Autodesk Fusion 360 part; units mm, degrees
note: some values were not read from the file. Set by a fixed rule: which sketch regions a step uses.
(part 2 of 6)
  line L1001 (386, 233.1906) -> (388, 234.3453)
  line L1002 (350.25, 210.9537) -> (352.25, 212.1084)
  line L1003 (360.5, 236.6547) -> (358.5, 237.8094)
  line L1004 (360.5, 236.6547) -> (358.5, 237.8094)
  line L1005 (378.5, 218.6547) -> (378.5, 216.3453)
  line L1006 (378.5, 245.6547) -> (378.5, 243.3453)
  line L1007 (378.5, 216.3453) -> (380.5, 215.1906)
  line L1008 (350.25, 206.5725) -> (348.25, 205.4178)
  line L1009 (355, 234.3453) -> (355, 236.6547)
  line L1010 (382.5, 243.3453) -> (382.5, 245.6547)
  line L1011 (391.5, 237.8094) -> (389.5, 236.6547)
  line L1012 (362, 236.6547) -> (362, 234.3453)
  line L1013 (388.75, 237.9537) -> (390.75, 239.1084)
  line L1014 (345.5, 207.3453) -> (347.5, 206.1906)
  line L1015 (379.75, 250.4178) -> (377.75, 251.5725)
  line L1016 (388.75, 233.5725) -> (386.75, 232.4178)
  line L1017 (347.5, 210.8094) -> (345.5, 209.6547)
  line L1018 (362, 236.6547) -> (362, 234.3453)
  line L1019 (377, 243.3453) -> (377, 245.6547)
  line L1020 (388, 236.6547) -> (386, 237.8094)
  line L1021 (381.25, 232.4178) -> (381.25, 230.1084)
  line L1022 (366, 227.6547) -> (364, 228.8094)
  line L1023 (382.5, 216.3453) -> (382.5, 218.6547)
  line L1024 (378.5, 245.6547) -> (378.5, 243.3453)
  line L1025 (388, 236.6547) -> (386, 237.8094)
  line L1026 (377, 243.3453) -> (377, 245.6547)
  line L1027 (358.5, 233.1906) -> (360.5, 234.3453)
  line L1028 (358.5, 237.8094) -> (356.5, 236.6547)
  line L1029 (389.5, 234.3453) -> (391.5, 233.1906)
  line L1030 (378.5, 243.3453) -> (380.5, 242.1906)
  line L1031 (382.5, 245.6547) -> (380.5, 246.8094)
  line L1032 (389.5, 234.3453) -> (391.5, 233.1906)
  line L1033 (350.25, 210.9537) -> (352.25, 212.1084)
  line L1034 (366.75, 224.5725) -> (364.75, 223.4178)
  line L1035 (358.5, 237.8094) -> (356.5, 236.6547)
  line L1036 (379.75, 241.4178) -> (377.75, 242.5725)
  line L1037 (388, 234.3453) -> (388, 236.6547)
  line L1038 (363.25, 230.1084) -> (363.25, 232.4178)
  line L1039 (351, 216.3453) -> (353, 215.1906)
  line L1040 (382.5, 245.6547) -> (380.5, 246.8094)
  line L1041 (359.25, 239.1084) -> (361.25, 237.9537)
  line L1042 (378.5436, 252.3202) -> (380.5, 251.1906)
  arc A23 (381.6602, 251.8605) -> (378.5436, 252.3202) centre (375, 217.5) ccw
  line L1043 (378.5436, 252.3202) -> (380.5, 251.1906)
  line L1044 (349.5, 216.3453) -> (349.5, 218.6547)
  line L1045 (377.75, 242.5725) -> (375.75, 241.4178)
  line L1046 (369.5, 237.8094) -> (367.5, 236.6547)
  line L1047 (380.5, 251.1906) -> (381.6602, 251.8605)
  line L1048 (375.75, 248.1084) -> (377.75, 246.9537)
  line L1049 (364.75, 239.1084) -> (366.75, 237.9537)
  line L1050 (367.5, 234.3453) -> (369.5, 233.1906)
  line L1051 (345.5, 209.6547) -> (345.5, 207.3453)
  line L1052 (347.5, 206.1906) -> (349.5, 207.3453)
  line L1053 (353.75, 239.1084) -> (355.75, 237.9537)
  line L1054 (375.75, 248.1084) -> (377.75, 246.9537)
  line L1055 (380.5, 246.8094) -> (378.5, 245.6547)
  line L1056 (353, 210.8094) -> (351, 209.6547)
  line L1057 (364, 233.1906) -> (366, 234.3453)
  line L1058 (356.5, 234.3453) -> (358.5, 233.1906)
  line L1059 (366.75, 242.5725) -> (364.75, 241.4178)
  line L1060 (368.75, 230.1084) -> (368.75, 232.4178)
  line L1061 (368.75, 230.1084) -> (368.75, 232.4178)
  line L1062 (366.75, 237.9537) -> (368.75, 239.1084)
  line L1063 (368.75, 232.4178) -> (366.75, 233.5725)
  line L1064 (353, 219.8094) -> (351, 218.6547)
  line L1065 (380.5, 242.1906) -> (382.5, 243.3453)
  line L1066 (360.5, 234.3453) -> (360.5, 236.6547)
  line L1067 (369.5, 228.8094) -> (367.5, 227.6547)
  line L1068 (348.25, 212.1084) -> (350.25, 210.9537)
  line L1069 (355.75, 237.9537) -> (357.75, 239.1084)
  line L1070 (390.75, 232.4178) -> (388.75, 233.5725)
  line L1071 (345.5, 218.6547) -> (345.5, 216.3453)
  line L1072 (367.5, 225.3453) -> (369.5, 224.1906)
  line L1073 (377.75, 251.5725) -> (375.75, 250.4178)
  line L1074 (368.75, 223.4178) -> (366.75, 224.5725)
  line L1075 (366, 236.6547) -> (364, 237.8094)
  line L1076 (390.75, 232.4178) -> (388.75, 233.5725)
  line L1077 (384, 234.3453) -> (386, 233.1906)
  line L1078 (346.75, 205.4178) -> (344.75, 206.5725)
  line L1079 (366.75, 237.9537) -> (368.75, 239.1084)
  line L1080 (350.25, 219.9537) -> (352.25, 221.1084)
  line L1081 (356.5, 236.6547) -> (356.5, 234.3453)
  line L1082 (366, 227.6547) -> (364, 228.8094)
  line L1083 (377.75, 242.5725) -> (375.75, 241.4178)
  line L1084 (352.25, 214.4178) -> (350.25, 215.5725)
  line L1085 (345.5, 216.3453) -> (347.5, 215.1906)
  line L1086 (361.25, 233.5725) -> (359.25, 232.4178)
  line L1087 (352.25, 214.4178) -> (350.25, 215.5725)
  line L1088 (352.25, 205.4178) -> (350.25, 206.5725)
  line L1089 (369.5, 237.8094) -> (367.5, 236.6547)
  line L1090 (360.5, 234.3453) -> (360.5, 236.6547)
  line L1091 (388.75, 237.9537) -> (390.75, 239.1084)
  line L1092 (364.75, 223.4178) -> (364.75, 221.1084)
  line L1093 (385.25, 241.4178) -> (383.25, 242.5725)
  line L1094 (349.5, 216.3453) -> (349.5, 218.6547)
  line L1095 (364, 242.1906) -> (366, 243.3453)
  line L1096 (366.75, 228.9537) -> (368.75, 230.1084)
  line L1097 (347.5, 219.8094) -> (345.5, 218.6547)
  line L1098 (364.75, 241.4178) -> (364.75, 239.1084)
  line L1099 (379.75, 250.4178) -> (377.75, 251.5725)
  line L1100 (368.75, 239.1084) -> (368.75, 241.4178)
  line L1101 (380.5, 237.8094) -> (378.5, 236.6547)
  line L1102 (345.5, 218.6547) -> (345.5, 216.3453)
  line L1103 (367.5, 234.3453) -> (369.5, 233.1906)
  line L1104 (347.5, 219.8094) -> (345.5, 218.6547)
  line L1105 (385.25, 241.4178) -> (383.25, 242.5725)
  line L1106 (366, 236.6547) -> (364, 237.8094)
  line L1107 (357.75, 239.1084) -> (357.75, 241.4178)
  line L1108 (357.75, 230.1084) -> (357.75, 232.4178)
  line L1109 (363.25, 239.1084) -> (363.25, 241.4178)
  line L1110 (346.75, 214.4178) -> (344.75, 215.5725)
  line L1111 (383.25, 242.5725) -> (381.25, 241.4178)
  line L1112 (367.5, 243.3453) -> (369.5, 242.1906)
  line L1113 (351, 216.3453) -> (353, 215.1906)
  line L1114 (369.5, 228.8094) -> (367.5, 227.6547)
  line L1115 (366.75, 228.9537) -> (368.75, 230.1084)
  line L1116 (368.75, 241.4178) -> (366.75, 242.5725)
  line L1117 (380.5, 233.1906) -> (382.5, 234.3453)
  line L1118 (377.75, 251.5725) -> (375.75, 250.4178)
  line L1119 (367.5, 225.3453) -> (369.5, 224.1906)
  line L1120 (347.5, 215.1906) -> (349.5, 216.3453)
  arc A24 (390.75, 248.756) -> (386.8045, 250.4493) centre (375, 217.5) ccw
  line L1121 (344.75, 219.9537) -> (346.75, 221.1084)
  line L1122 (347.5, 215.1906) -> (349.5, 216.3453)
  line L1123 (363.25, 239.1084) -> (363.25, 241.4178)
  line L1124 (364.75, 230.1084) -> (366.75, 228.9537)
  line L1125 (359.25, 232.4178) -> (359.25, 230.1084)
  line L1126 (359.25, 232.4178) -> (359.25, 230.1084)
  line L1127 (350.25, 215.5725) -> (348.25, 214.4178)
  line L1128 (353.75, 232.4178) -> (353.75, 230.1084)
  line L1129 (356.5, 236.6547) -> (356.5, 234.3453)
  line L1130 (377.75, 237.9537) -> (379.75, 239.1084)
  line L1131 (359.25, 241.4178) -> (359.25, 239.1084)
  line L1132 (383.25, 242.5725) -> (381.25, 241.4178)
  line L1133 (349.5, 218.6547) -> (347.5, 219.8094)
  line L1134 (363.25, 221.1084) -> (363.25, 223.4178)
  line L1135 (364.75, 232.4178) -> (364.75, 230.1084)
  line L1136 (350.25, 215.5725) -> (348.25, 214.4178)
  line L1137 (381.25, 232.4178) -> (381.25, 230.1084)
  line L1138 (364, 224.1906) -> (366, 225.3453)
  line L1139 (344.75, 219.9537) -> (346.75, 221.1084)
  line L1140 (366.75, 224.5725) -> (364.75, 223.4178)
  line L1141 (364.75, 241.4178) -> (364.75, 239.1084)
  line L1142 (377, 252.3453) -> (377, 252.4428)
  line L1143 (367.5, 245.6547) -> (367.5, 243.3453)
  line L1144 (353.75, 232.4178) -> (353.75, 230.1084)
  arc A25 (381.6602, 251.8605) -> (378.5436, 252.3202) centre (375, 217.5) ccw
  line L1145 (366.75, 242.5725) -> (364.75, 241.4178)
  line L1146 (357.75, 230.1084) -> (357.75, 232.4178)
  line L1147 (366.75, 233.5725) -> (364.75, 232.4178)
  line L1148 (348.25, 221.1084) -> (350.25, 219.9537)
  line L1149 (386.8045, 250.4493) -> (386.75, 250.4178)
  line L1150 (368.75, 241.4178) -> (366.75, 242.5725)
  line L1151 (377, 234.3453) -> (377, 236.6547)
  line L1152 (368.75, 239.1084) -> (368.75, 241.4178)
  line L1153 (375.75, 239.1084) -> (377.75, 237.9537)
  line L1154 (346.75, 223.4178) -> (344.75, 224.5725)
  line L1155 (367.5, 245.6547) -> (367.5, 243.3453)
  line L1156 (364.75, 250.4178) -> (364.75, 248.1084)
  line L1157 (363.25, 230.1084) -> (363.25, 232.4178)
  line L1158 (350.25, 219.9537) -> (352.25, 221.1084)
  line L1159 (355, 236.6547) -> (353, 237.8094)
  line L1160 (377.75, 233.5725) -> (375.75, 232.4178)
  line L1161 (364.75, 239.1084) -> (366.75, 237.9537)
  line L1162 (355, 236.6547) -> (353, 237.8094)
  line L1163 (368.75, 221.1084) -> (368.75, 223.4178)
  line L1164 (390.75, 230.1084) -> (390.75, 232.4178)
  line L1165 (366, 243.3453) -> (366, 245.6547)
  line L1166 (378.5, 236.6547) -> (378.5, 234.3453)
  line L1167 (364.75, 232.4178) -> (364.75, 230.1084)
  line L1168 (348.25, 221.1084) -> (350.25, 219.9537)
  line L1169 (353, 219.8094) -> (351, 218.6547)
  line L1170 (353, 233.1906) -> (355, 234.3453)
  line L1171 (351, 218.6547) -> (351, 216.3453)
  line L1172 (355, 227.6547) -> (353, 228.8094)
  line L1173 (368.75, 223.4178) -> (366.75, 224.5725)
  line L1174 (351, 218.6547) -> (351, 216.3453)
  line L1175 (377.75, 233.5725) -> (375.75, 232.4178)
  line L1176 (345.5, 216.3453) -> (347.5, 215.1906)
  line L1177 (359.25, 248.756) -> (359.25, 248.1084)
  line L1178 (366, 225.3453) -> (366, 227.6547)
  line L1179 (380.5, 233.1906) -> (382.5, 234.3453)
  line L1180 (348.25, 230.1084) -> (350.25, 228.9537)
  line L1181 (359.25, 248.756) -> (359.25, 248.1084)
  line L1182 (377, 234.3453) -> (377, 236.6547)
  line L1183 (380.5, 251.1906) -> (381.6602, 251.8605)
  line L1184 (368.75, 248.1084) -> (368.75, 250.4178)
  line L1185 (382.5, 236.6547) -> (380.5, 237.8094)
  line L1186 (346.75, 214.4178) -> (344.75, 215.5725)
  line L1187 (383.25, 237.9537) -> (385.25, 239.1084)
  line L1188 (353, 224.1906) -> (355, 225.3453)
  line L1189 (377.75, 237.9537) -> (379.75, 239.1084)
  line L1190 (364, 233.1906) -> (366, 234.3453)
  line L1191 (382.5, 234.3453) -> (382.5, 236.6547)
  line L1192 (366, 243.3453) -> (366, 245.6547)
  line L1193 (366.75, 233.5725) -> (364.75, 232.4178)
  line L1194 (375.75, 232.4178) -> (375.75, 230.1084)
  line L1195 (364.75, 230.1084) -> (366.75, 228.9537)
  line L1196 (368.3398, 251.8605) -> (369.5, 251.1906)
  line L1197 (364, 242.1906) -> (366, 243.3453)
  line L1198 (368.75, 232.4178) -> (366.75, 233.5725)
  line L1199 (352.25, 223.4178) -> (350.25, 224.5725)
  line L1200 (386.75, 232.4178) -> (386.75, 230.1084)
  line L1201 (367.5, 227.6547) -> (367.5, 225.3453)
  line L1202 (367.5, 243.3453) -> (369.5, 242.1906)
  line L1203 (364, 224.1906) -> (366, 225.3453)
  line L1204 (353, 233.1906) -> (355, 234.3453)
  line L1205 (379.75, 232.4178) -> (377.75, 233.5725)
  line L1206 (366, 225.3453) -> (366, 227.6547)
  line L1207 (382.5, 234.3453) -> (382.5, 236.6547)
  line L1208 (349.5, 218.6547) -> (347.5, 219.8094)
  line L1209 (385.25, 230.1084) -> (385.25, 232.4178)
  line L1210 (363.25, 250.4178) -> (363.1955, 250.4493)
  arc A26 (354.558, 245.9099) -> (351.2448, 243.2039) centre (375, 217.5) ccw
  line L1211 (356.5, 243.3453) -> (358.5, 242.1906)
  line L1212 (379.75, 232.4178) -> (377.75, 233.5725)
  line L1213 (363.25, 221.1084) -> (363.25, 223.4178)
  line L1214 (368.75, 221.1084) -> (368.75, 223.4178)
  arc A27 (350.4572, 242.4529) -> (348.25, 240.0707) centre (375, 217.5) ccw
  line L1215 (357.75, 241.4178) -> (355.75, 242.5725)
  line L1216 (351, 227.6547) -> (351, 225.3453)
  line L1217 (385.25, 232.4178) -> (383.25, 233.5725)
  line L1218 (382.5, 236.6547) -> (380.5, 237.8094)
  line L1219 (356.5, 245.6547) -> (356.5, 243.3453)
  line L1220 (378.5, 236.6547) -> (378.5, 234.3453)
  line L1221 (355, 245.6547) -> (354.558, 245.9099)
  line L1222 (364.75, 223.4178) -> (364.75, 221.1084)
  line L1223 (353, 228.8094) -> (351, 227.6547)
  line L1224 (361.25, 242.5725) -> (359.25, 241.4178)
  line L1225 (405.25, 210.9537) -> (407.25, 212.1084)
  line L1226 (409.917, 215.0916) -> (408.75, 214.4178)
  line L1227 (405.25, 215.5725) -> (403.25, 214.4178)
  line L1228 (403.25, 214.4178) -> (403.25, 212.1084)
  line L1229 (408, 215.1906) -> (409.9806, 216.3341)
  line L1230 (409.211, 210.1102) -> (408, 210.8094)
  line L1231 (407.25, 212.1084) -> (407.25, 214.4178)
  line L1232 (405.25, 215.5725) -> (403.25, 214.4178)
  line L1233 (407.25, 214.4178) -> (405.25, 215.5725)
  arc A28 (409.5109, 211.6691) -> (409.917, 215.0916) centre (375, 217.5) ccw
  line L1234 (408, 210.8094) -> (406, 209.6547)
  line L1235 (407.25, 214.4178) -> (405.25, 215.5725)
  line L1236 (408, 215.1906) -> (409.9806, 216.3341)
  line L1237 (407.25, 221.1084) -> (407.25, 223.4178)
  line L1238 (375, 242.1906) -> (377, 243.3453)
  line L1239 (407.25, 223.4178) -> (405.25, 224.5725)
  line L1240 (404.5, 216.3453) -> (404.5, 218.6547)
  line L1241 (405.25, 219.9537) -> (407.25, 221.1084)
  line L1242 (409.4268, 223.8086) -> (408.75, 223.4178)
  line L1243 (408, 219.8094) -> (406, 218.6547)
  line L1244 (403.25, 223.4178) -> (403.25, 221.1084)
  line L1245 (406, 225.3453) -> (408, 224.1906)
  line L1246 (405.25, 224.5725) -> (403.25, 223.4178)
  line L1247 (408.75, 223.4178) -> (408.75, 221.1084)
  line L1248 (407.25, 221.1084) -> (407.25, 223.4178)
  line L1249 (408.75, 221.1084) -> (409.8747, 220.4591)
  line L1250 (407.25, 223.4178) -> (405.25, 224.5725)
  line L1251 (405.25, 219.9537) -> (407.25, 221.1084)
  line L1252 (403.25, 223.4178) -> (403.25, 221.1084)
  line L1253 (408, 219.8094) -> (406, 218.6547)
  line L1254 (408.75, 223.4178) -> (408.75, 221.1084)
  line L1255 (403.25, 221.1084) -> (405.25, 219.9537)
  line L1256 (409.4268, 223.8086) -> (408.75, 223.4178)
  arc A29 (410, 217.5) -> (409.9806, 218.6659) centre (375, 217.5) ccw
  arc A30 (410, 217.5) -> (409.9806, 218.6659) centre (375, 217.5) ccw
  line L1257 (403.25, 221.1084) -> (405.25, 219.9537)
  line L1258 (409.9806, 218.6659) -> (408, 219.8094)
  line L1259 (409.9806, 218.6659) -> (408, 219.8094)
  line L1260 (408.75, 221.1084) -> (409.8747, 220.4591)
  line L1261 (405.25, 224.5725) -> (403.25, 223.4178)
  arc A31 (409.8747, 220.4591) -> (409.4268, 223.8086) centre (375, 217.5) ccw
  line L1262 (408, 224.1906) -> (409.211, 224.8898)
  line L1263 (406, 216.3453) -> (408, 215.1906)
  arc A32 (409.9806, 216.3341) -> (410, 217.5) centre (375, 217.5) ccw
  line L1264 (406, 216.3453) -> (408, 215.1906)
  line L1265 (406, 218.6547) -> (406, 216.3453)
  line L1266 (406, 225.3453) -> (408, 224.1906)
  line L1267 (406, 218.6547) -> (406, 216.3453)
  line L1268 (404.5, 216.3453) -> (404.5, 218.6547)
  line L1269 (408, 224.1906) -> (409.211, 224.8898)
  arc A33 (409.9806, 216.3341) -> (410, 217.5) centre (375, 217.5) ccw
  arc A34 (392.25, 187.0461) -> (394.4942, 188.4315) centre (375, 217.5) ccw
  line L1270 (394.4942, 188.4315) -> (394.25, 188.5725)
  line L1271 (394.25, 188.5725) -> (392.25, 187.4178)
  arc A35 (392.25, 187.0461) -> (394.4942, 188.4315) centre (375, 217.5) ccw
  line L1272 (394.25, 188.5725) -> (392.25, 187.4178)
  line L1273 (394.4942, 188.4315) -> (394.25, 188.5725)
  line L1274 (386.75, 194.1084) -> (388.75, 192.9537)
  line L1275 (399.5428, 242.4529) -> (397.75, 241.4178)
  line L1276 (381.25, 205.4178) -> (381.25, 203.1084)
  line L1277 (362, 216.3453) -> (364, 215.1906)
  line L1278 (396.25, 230.1084) -> (396.25, 232.4178)
  line L1279 (368.75, 212.1084) -> (368.75, 214.4178)
  line L1280 (371.5, 225.3453) -> (371.5, 227.6547)
  line L1281 (388, 198.3453) -> (388, 200.6547)
  line L1282 (399, 227.6547) -> (397, 228.8094)
  line L1283 (386, 197.1906) -> (388, 198.3453)
  line L1284 (397, 242.1906) -> (398.7552, 243.2039)
  arc A36 (398.7552, 243.2039) -> (395.442, 245.9099) centre (375, 217.5) ccw
  line L1285 (372.25, 197.5725) -> (370.25, 196.4178)
  line L1286 (386, 201.8094) -> (384, 200.6547)
  line L1287 (386.75, 194.1084) -> (388.75, 192.9537)
  line L1288 (372.25, 224.5725) -> (370.25, 223.4178)
  line L1289 (392.25, 196.4178) -> (392.25, 194.1084)
  line L1290 (399.5428, 242.4529) -> (397.75, 241.4178)
  line L1291 (393.5, 243.3453) -> (393.5, 245.6547)
  line L1292 (375, 192.8094) -> (373, 191.6547)
  line L1293 (372.25, 233.5725) -> (370.25, 232.4178)
  line L1294 (371.5, 225.3453) -> (371.5, 227.6547)
  line L1295 (374.25, 196.4178) -> (372.25, 197.5725)
  line L1296 (395.442, 245.9099) -> (395, 245.6547)
  line L1297 (395, 245.6547) -> (395, 243.3453)
  line L1298 (396.25, 230.1084) -> (396.25, 232.4178)
  line L1299 (389.5, 200.6547) -> (389.5, 198.3453)
  line L1300 (390.75, 196.4178) -> (388.75, 197.5725)
  line L1301 (401.75, 232.4178) -> (399.75, 233.5725)
  line L1302 (390.75, 239.1084) -> (390.75, 241.4178)
  line L1303 (395.442, 245.9099) -> (395, 245.6547)
  line L1304 (370.25, 230.1084) -> (372.25, 228.9537)
  line L1305 (392.25, 205.4178) -> (392.25, 203.1084)
  line L1306 (402.5, 233.1906) -> (404.5, 234.3453)
  line L1307 (370.25, 194.1084) -> (372.25, 192.9537)
  line L1308 (399, 227.6547) -> (397, 228.8094)
  line L1309 (395, 245.6547) -> (395, 243.3453)
  line L1310 (389.5, 198.3453) -> (391.5, 197.1906)
  line L1311 (372.25, 201.9537) -> (374.25, 203.1084)
  line L1312 (401.75, 232.4178) -> (399.75, 233.5725)
  line L1313 (353.75, 223.4178) -> (353.75, 221.1084)
  line L1314 (370.25, 196.4178) -> (370.25, 194.1084)
  line L1315 (396.25, 241.4178) -> (394.25, 242.5725)
  line L1316 (394.25, 228.9537) -> (396.25, 230.1084)
  line L1317 (372.25, 197.5725) -> (370.25, 196.4178)
  line L1318 (397.75, 230.1084) -> (399.75, 228.9537)
  line L1319 (395, 234.3453) -> (397, 233.1906)
  line L1320 (375, 201.8094) -> (373, 200.6547)
  line L1321 (404.1665, 236.8473) -> (402.5, 237.8094)
  line L1322 (373, 234.3453) -> (375, 233.1906)
  line L1323 (384, 198.3453) -> (386, 197.1906)
  line L1324 (375, 228.8094) -> (373, 227.6547)
  line L1325 (395, 243.3453) -> (397, 242.1906)
  line L1326 (363.25, 205.4178) -> (361.25, 206.5725)
  line L1327 (372.25, 228.9537) -> (374.25, 230.1084)
  line L1328 (397, 242.1906) -> (398.7552, 243.2039)
  line L1329 (395, 243.3453) -> (397, 242.1906)
  line L1330 (370.25, 230.1084) -> (372.25, 228.9537)
  line L1331 (397.75, 230.1084) -> (399.75, 228.9537)
  line L1332 (385.25, 203.1084) -> (385.25, 205.4178)
  line L1333 (370.25, 232.4178) -> (370.25, 230.1084)
  line L1334 (392.25, 196.4178) -> (392.25, 194.1084)
  line L1335 (397.75, 232.4178) -> (397.75, 230.1084)
  line L1336 (363.25, 241.4178) -> (361.25, 242.5725)
  line L1337 (360.5, 189.3453) -> (360.5, 191.6547)
  line L1338 (366.75, 206.5725) -> (364.75, 205.4178)
  line L1339 (359.25, 203.1084) -> (361.25, 201.9537)
  line L1340 (391.5, 242.1906) -> (393.5, 243.3453)
  line L1341 (342, 228.8094) -> (341.8476, 228.7214)
  line L1342 (395, 209.6547) -> (395, 207.3453)
  line L1343 (395, 209.6547) -> (395, 207.3453)
  line L1344 (406, 209.6547) -> (406, 207.3453)
  line L1345 (340.789, 224.8898) -> (342, 224.1906)
  line L1346 (372.25, 206.5725) -> (370.25, 205.4178)
  line L1347 (342, 228.8094) -> (341.8476, 228.7214)
  line L1348 (393.5, 207.3453) -> (393.5, 209.6547)
  line L1349 (342, 219.8094) -> (340.0194, 218.6659)
  line L1350 (359.25, 194.1084) -> (361.25, 192.9537)
  line L1351 (399, 207.3453) -> (399, 209.6547)
  line L1352 (364, 237.8094) -> (362, 236.6547)
  line L1353 (373, 209.6547) -> (373, 207.3453)
  arc A37 (341.8476, 228.7214) -> (340.789, 224.8898) centre (375, 217.5) ccw
  line L1354 (363.25, 232.4178) -> (361.25, 233.5725)
  line L1355 (341.25, 214.4178) -> (340.083, 215.0916)
  arc A38 (341.8476, 228.7214) -> (340.789, 224.8898) centre (375, 217.5) ccw
  line L1356 (361.25, 192.9537) -> (363.25, 194.1084)
  line L1357 (404.5, 207.3453) -> (404.5, 209.6547)
  line L1358 (361.25, 201.9537) -> (363.25, 203.1084)
  line L1359 (373, 209.6547) -> (373, 207.3453)
  line L1360 (394.25, 215.5725) -> (392.25, 214.4178)
  line L1361 (342, 215.1906) -> (344, 216.3453)
  line L1362 (400.5, 209.6547) -> (400.5, 207.3453)
  line L1363 (393.5, 236.6547) -> (391.5, 237.8094)
  arc A39 (340.789, 210.1102) -> (341.8476, 206.2786) centre (375, 217.5) ccw
  line L1364 (364.75, 187.4178) -> (364.75, 185.1084)
  line L1365 (362, 225.3453) -> (364, 224.1906)
  line L1366 (392.25, 212.1084) -> (394.25, 210.9537)
  line L1367 (368.75, 187.4178) -> (366.75, 188.5725)
  line L1368 (369.5, 206.1906) -> (371.5, 207.3453)
  line L1369 (356.5, 191.6547) -> (356.5, 189.3453)
  line L1370 (364.75, 185.1084) -> (366.75, 183.9537)
  line L1371 (393.5, 218.6547) -> (391.5, 219.8094)
  arc A40 (359.25, 186.244) -> (362.6388, 184.7555) centre (375, 217.5) ccw
  line L1372 (363.25, 196.4178) -> (361.25, 197.5725)
  line L1373 (344, 209.6547) -> (342, 210.8094)
  line L1374 (400.5, 209.6547) -> (400.5, 207.3453)
  line L1375 (341.25, 223.4178) -> (340.5732, 223.8086)
  line L1376 (394.25, 242.5725) -> (392.25, 241.4178)
  line L1377 (340.1253, 220.4591) -> (341.25, 221.1084)
  line L1378 (341.25, 212.1084) -> (341.25, 214.4178)
  line L1379 (393.5, 227.6547) -> (391.5, 228.8094)
  line L1380 (344, 218.6547) -> (342, 219.8094)
  line L1381 (364.75, 185.1084) -> (366.75, 183.9537)
  arc A41 (408.1524, 206.2786) -> (409.211, 210.1102) centre (375, 217.5) ccw
  line L1382 (344, 216.3453) -> (344, 218.6547)
  line L1383 (375, 210.8094) -> (373, 209.6547)
  line L1384 (363.25, 185.1084) -> (363.25, 187.4178)
  line L1385 (344, 216.3453) -> (344, 218.6547)
  line L1386 (364, 228.8094) -> (362, 227.6547)
  line L1387 (366.75, 188.5725) -> (364.75, 187.4178)
  line L1388 (363.25, 232.4178) -> (361.25, 233.5725)
  line L1389 (342.75, 214.4178) -> (342.75, 212.1084)
  line L1390 (399, 207.3453) -> (399, 209.6547)
  line L1391 (391.5, 206.1906) -> (393.5, 207.3453)
  line L1392 (344, 218.6547) -> (342, 219.8094)
  line L1393 (364.75, 212.1084) -> (366.75, 210.9537)
  line L1394 (406, 209.6547) -> (406, 207.3453)
  line L1395 (358.5, 188.1906) -> (360.5, 189.3453)
  line L1396 (373, 191.6547) -> (373, 189.3453)
  line L1397 (357.75, 187.0461) -> (357.75, 187.4178)
  line L1398 (364, 188.1906) -> (366, 189.3453)
  line L1399 (368.75, 187.4178) -> (366.75, 188.5725)
  line L1400 (355, 189.3453) -> (355, 191.6547)
  line L1401 (367.5, 209.6547) -> (367.5, 207.3453)
  line L1402 (361.25, 228.9537) -> (363.25, 230.1084)
  line L1403 (366, 207.3453) -> (366, 209.6547)
  line L1404 (363.25, 185.1084) -> (363.25, 187.4178)
  line L1405 (366.75, 210.9537) -> (368.75, 212.1084)
  line L1406 (392.25, 194.1084) -> (394.25, 192.9537)
  line L1407 (342.75, 214.4178) -> (342.75, 212.1084)
  line L1408 (355.75, 188.5725) -> (355.5058, 188.4315)
  line L1409 (354.558, 189.0901) -> (355, 189.3453)
  line L1410 (341.25, 214.4178) -> (340.083, 215.0916)
  line L1411 (391.5, 215.1906) -> (393.5, 216.3453)
  line L1412 (393.5, 227.6547) -> (391.5, 228.8094)
  line L1413 (366.75, 206.5725) -> (364.75, 205.4178)
  line L1414 (368.75, 185.1084) -> (368.75, 187.4178)
  line L1415 (366, 189.3453) -> (366, 191.6547)
  line L1416 (394.25, 197.5725) -> (392.25, 196.4178)
  line L1417 (340.1253, 220.4591) -> (341.25, 221.1084)
  line L1418 (393.5, 207.3453) -> (393.5, 209.6547)
  line L1419 (394.25, 233.5725) -> (392.25, 232.4178)
  line L1420 (362, 189.3453) -> (364, 188.1906)
  line L1421 (393.5, 236.6547) -> (391.5, 237.8094)
  line L1422 (355, 189.3453) -> (355, 191.6547)
  line L1423 (340.0194, 216.3341) -> (342, 215.1906)
  arc A42 (408.1524, 206.2786) -> (409.211, 210.1102) centre (375, 217.5) ccw
  line L1424 (367.5, 209.6547) -> (367.5, 207.3453)
  line L1425 (362, 207.3453) -> (364, 206.1906)
  line L1426 (356.5, 191.6547) -> (356.5, 189.3453)
  line L1427 (362.6388, 184.7555) -> (363.25, 185.1084)
  line L1428 (362, 191.6547) -> (362, 189.3453)
  line L1429 (368.75, 205.4178) -> (366.75, 206.5725)
  line L1430 (342, 215.1906) -> (344, 216.3453)
  line L1431 (361.25, 210.9537) -> (363.25, 212.1084)
  line L1432 (366, 189.3453) -> (366, 191.6547)
  line L1433 (341.25, 212.1084) -> (341.25, 214.4178)
  line L1434 (364.75, 212.1084) -> (366.75, 210.9537)
  line L1435 (364, 206.1906) -> (366, 207.3453)
  line L1436 (360.5, 189.3453) -> (360.5, 191.6547)
  line L1437 (342, 219.8094) -> (340.0194, 218.6659)
  line L1438 (340.0194, 216.3341) -> (342, 215.1906)
  line L1439 (357.75, 187.0461) -> (357.75, 187.4178)
  line L1440 (366, 209.6547) -> (364, 210.8094)
  line L1441 (363.25, 223.4178) -> (361.25, 224.5725)
  line L1442 (355.75, 188.5725) -> (355.5058, 188.4315)
  line L1443 (364, 188.1906) -> (366, 189.3453)
  arc A43 (340.0194, 218.6659) -> (340, 217.5) centre (375, 217.5) ccw
  line L1444 (353, 197.1906) -> (355, 198.3453)
  line L1445 (362, 189.3453) -> (364, 188.1906)
  line L1446 (362, 234.3453) -> (364, 233.1906)
  line L1447 (356.5, 189.3453) -> (358.5, 188.1906)
  arc A44 (340.0194, 218.6659) -> (340, 217.5) centre (375, 217.5) ccw
  line L1448 (356.5, 189.3453) -> (358.5, 188.1906)
  line L1449 (368.75, 205.4178) -> (366.75, 206.5725)
  line L1450 (355, 191.6547) -> (353, 192.8094)
  line L1451 (393.5, 225.3453) -> (393.5, 227.6547)
  line L1452 (392.25, 230.1084) -> (394.25, 228.9537)
  line L1453 (366.75, 188.5725) -> (364.75, 187.4178)
  arc A45 (404.5, 236.3348) -> (404.1665, 236.8473) centre (375, 217.5) ccw
  line L1454 (405.25, 233.5725) -> (403.25, 232.4178)
  line L1455 (399, 225.3453) -> (399, 227.6547)
  arc A46 (404.5, 236.3348) -> (404.1665, 236.8473) centre (375, 217.5) ccw
  line L1456 (357.75, 194.1084) -> (357.75, 196.4178)
  line L1457 (369.5, 210.8094) -> (367.5, 209.6547)
  line L1458 (355, 200.6547) -> (353, 201.8094)
  line L1459 (371.5, 189.3453) -> (371.5, 191.6547)
  line L1460 (359.25, 187.4178) -> (359.25, 186.244)
  arc A47 (368.3398, 183.1395) -> (371.4564, 182.6798) centre (375, 217.5) ccw
  arc A48 (409.211, 224.8898) -> (408.1524, 228.7214) centre (375, 217.5) ccw
  line L1461 (351, 200.6547) -> (351, 198.3453)
  line L1462 (369.5, 183.8094) -> (368.3398, 183.1395)
  line L1463 (369.5, 188.1906) -> (371.5, 189.3453)
  line L1464 (356.5, 200.6547) -> (356.5, 198.3453)
  line L1465 (407.25, 230.1084) -> (407.25, 231.0992)
  line L1466 (355, 191.6547) -> (353, 192.8094)
  line L1467 (364.75, 187.4178) -> (364.75, 185.1084)
  line L1468 (361.25, 246.9537) -> (363.25, 248.1084)
  line L1469 (371.4564, 182.6798) -> (369.5, 183.8094)
  line L1470 (400.5, 227.6547) -> (400.5, 225.3453)
  line L1471 (367.5, 189.3453) -> (369.5, 188.1906)
  line L1472 (392.25, 212.1084) -> (394.25, 210.9537)
  line L1473 (361.25, 237.9537) -> (363.25, 239.1084)
  line L1474 (356.5, 198.3453) -> (358.5, 197.1906)
  line L1475 (360.5, 198.3453) -> (360.5, 200.6547)
  line L1476 (350.25, 192.9537) -> (352.25, 194.1084)
  line L1477 (388.75, 219.9537) -> (390.75, 221.1084)
  line L1478 (357.75, 187.4178) -> (355.75, 188.5725)
  line L1479 (366.75, 210.9537) -> (368.75, 212.1084)
  line L1480 (364, 206.1906) -> (366, 207.3453)
  line L1481 (366.75, 183.9537) -> (368.75, 185.1084)
  line L1482 (400.5, 227.6547) -> (400.5, 225.3453)
  line L1483 (367.5, 207.3453) -> (369.5, 206.1906)
  line L1484 (399, 225.3453) -> (399, 227.6547)
  arc A49 (363.1955, 250.4493) -> (359.25, 248.756) centre (375, 217.5) ccw
  line L1485 (355, 200.6547) -> (353, 201.8094)
  line L1486 (366, 207.3453) -> (366, 209.6547)
  line L1487 (367.5, 207.3453) -> (369.5, 206.1906)
  line L1488 (369.5, 210.8094) -> (367.5, 209.6547)
  line L1489 (353, 197.1906) -> (355, 198.3453)
  line L1490 (358.5, 188.1906) -> (360.5, 189.3453)
  line L1491 (357.75, 187.4178) -> (355.75, 188.5725)
  line L1492 (366.75, 183.9537) -> (368.75, 185.1084)
  line L1493 (359.25, 187.4178) -> (359.25, 186.244)
  line L1494 (393.5, 225.3453) -> (393.5, 227.6547)
  line L1495 (367.5, 191.6547) -> (367.5, 189.3453)
  line L1496 (368.75, 185.1084) -> (368.75, 187.4178)
  line L1497 (354.558, 189.0901) -> (355, 189.3453)
  line L1498 (366, 209.6547) -> (364, 210.8094)
  line L1499 (362.6388, 184.7555) -> (363.25, 185.1084)
  line L1500 (351, 200.6547) -> (351, 198.3453)
  line L1501 (408, 228.8094) -> (406, 227.6547)
  line L1502 (371.4564, 182.6798) -> (369.5, 183.8094)
  line L1503 (360.5, 200.6547) -> (358.5, 201.8094)
  line L1504 (373, 191.6547) -> (373, 189.3453)
  line L1505 (377.75, 219.9537) -> (379.75, 221.1084)
  line L1506 (360.5, 191.6547) -> (358.5, 192.8094)
  arc A50 (348.25, 194.9293) -> (349.7943, 193.2169) centre (375, 217.5) ccw
  line L1507 (358.5, 197.1906) -> (360.5, 198.3453)
  line L1508 (353, 192.8094) -> (351.2448, 191.7961)
  line L1509 (388.75, 219.9537) -> (390.75, 221.1084)
  line L1510 (364, 210.8094) -> (362, 209.6547)
  line L1511 (355.75, 197.5725) -> (353.75, 196.4178)
  line L1512 (353, 201.8094) -> (351, 200.6547)
  line L1513 (404.5, 234.3453) -> (404.5, 236.3348)
  line L1514 (349.5, 198.3453) -> (349.5, 200.6547)
  line L1515 (369.5, 183.8094) -> (368.3398, 183.1395)
  line L1516 (353.75, 196.4178) -> (353.75, 194.1084)
  line L1517 (405.25, 233.5725) -> (403.25, 232.4178)
  line L1518 (353.75, 203.1084) -> (355.75, 201.9537)
  line L1519 (403.25, 232.4178) -> (403.25, 230.1084)
  line L1520 (355, 198.3453) -> (355, 200.6547)
  line L1521 (351, 198.3453) -> (353, 197.1906)
  line L1522 (360.5, 198.3453) -> (360.5, 200.6547)
  arc A51 (368.3398, 183.1395) -> (371.4564, 182.6798) centre (375, 217.5) ccw
  line L1523 (406.4359, 232.8879) -> (405.25, 233.5725)
  line L1524 (361.25, 219.9537) -> (363.25, 221.1084)
  line L1525 (406.4359, 232.8879) -> (405.25, 233.5725)
  line L1526 (357.75, 196.4178) -> (355.75, 197.5725)
  line L1527 (356.5, 200.6547) -> (356.5, 198.3453)
  line L1528 (353, 192.8094) -> (351.2448, 191.7961)
  line L1529 (363.25, 214.4178) -> (361.25, 215.5725)
  line L1530 (377.75, 219.9537) -> (379.75, 221.1084)
  line L1531 (352.25, 194.1084) -> (352.25, 196.4178)
  line L1532 (408.1524, 228.7214) -> (408, 228.8094)
  line L1533 (348.25, 196.4178) -> (348.25, 194.9293)
  line L1534 (356.5, 198.3453) -> (358.5, 197.1906)
  line L1535 (364, 246.8094) -> (362, 245.6547)
  line L1536 (358.5, 201.8094) -> (356.5, 200.6547)
  arc A52 (409.211, 224.8898) -> (408.1524, 228.7214) centre (375, 217.5) ccw
  arc A53 (363.1955, 250.4493) -> (359.25, 248.756) centre (375, 217.5) ccw
  line L1537 (371.5, 189.3453) -> (371.5, 191.6547)
  line L1538 (404.5, 234.3453) -> (404.5, 236.3348)
  line L1539 (369.5, 188.1906) -> (371.5, 189.3453)
  line L1540 (353.75, 194.1084) -> (355.75, 192.9537)
  line L1541 (367.5, 189.3453) -> (369.5, 188.1906)
  line L1542 (353, 201.8094) -> (351, 200.6547)
  line L1543 (353.75, 196.4178) -> (353.75, 194.1084)
  line L1544 (352.25, 194.1084) -> (352.25, 196.4178)
  line L1545 (355.75, 201.9537) -> (357.75, 203.1084)
  line L1546 (408.1524, 228.7214) -> (408, 228.8094)
  line L1547 (395, 227.6547) -> (395, 225.3453)
  line L1548 (350.25, 192.9537) -> (352.25, 194.1084)
  line L1549 (406, 227.6547) -> (406, 225.3453)
  arc A54 (348.25, 194.9293) -> (349.7943, 193.2169) centre (375, 217.5) ccw
  line L1550 (351, 198.3453) -> (353, 197.1906)
  line L1551 (348.25, 196.4178) -> (348.25, 194.9293)
  line L1552 (404.5, 225.3453) -> (404.5, 227.6547)
  line L1553 (374.25, 214.4178) -> (372.25, 215.5725)
  line L1554 (360.5, 200.6547) -> (358.5, 201.8094)
  arc A55 (407.25, 231.0992) -> (406.4359, 232.8879) centre (375, 217.5) ccw
  line L1555 (403.25, 230.1084) -> (405.25, 228.9537)
  line L1556 (364, 246.8094) -> (362, 245.6547)
  line L1557 (370.25, 221.1084) -> (372.25, 219.9537)
  line L1558 (403.25, 230.1084) -> (405.25, 228.9537)
  line L1559 (386.75, 221.1084) -> (388.75, 219.9537)
  line L1560 (373, 216.3453) -> (375, 215.1906)
  line L1561 (375.75, 221.1084) -> (377.75, 219.9537)
  line L1562 (388.75, 197.5725) -> (386.75, 196.4178)
  line L1563 (372.25, 219.9537) -> (374.25, 221.1084)
  line L1564 (362, 191.6547) -> (362, 189.3453)
  line L1565 (358.5, 192.8094) -> (356.5, 191.6547)
  line L1566 (373, 198.3453) -> (375, 197.1906)
  line L1567 (358.5, 197.1906) -> (360.5, 198.3453)
  line L1568 (371.5, 216.3453) -> (371.5, 218.6547)
  line L1569 (355, 198.3453) -> (355, 200.6547)
  line L1570 (388.75, 192.9537) -> (390.75, 194.1084)
  line L1571 (407.25, 230.1084) -> (407.25, 231.0992)
  line L1572 (375, 219.8094) -> (373, 218.6547)
  line L1573 (355.75, 201.9537) -> (357.75, 203.1084)
  line L1574 (367.5, 191.6547) -> (367.5, 189.3453)
  line L1575 (352.25, 196.4178) -> (350.25, 197.5725)
  line L1576 (359.25, 196.4178) -> (359.25, 194.1084)
  line L1577 (373, 218.6547) -> (373, 216.3453)
  line L1578 (406, 227.6547) -> (406, 225.3453)
  line L1579 (348.25, 203.1084) -> (350.25, 201.9537)
  line L1580 (404.5, 225.3453) -> (404.5, 227.6547)
  line L1581 (371.5, 216.3453) -> (371.5, 218.6547)
  line L1582 (370.25, 203.1084) -> (372.25, 201.9537)
  line L1583 (388, 198.3453) -> (388, 200.6547)
  line L1584 (348.25, 203.1084) -> (350.25, 201.9537)
  line L1585 (355.75, 192.9537) -> (357.75, 194.1084)
  line L1586 (390.75, 196.4178) -> (388.75, 197.5725)
  line L1587 (405.25, 228.9537) -> (407.25, 230.1084)
  line L1588 (373, 218.6547) -> (373, 216.3453)
  line L1589 (349.7943, 193.2169) -> (350.25, 192.9537)
  line L1590 (372.25, 192.9537) -> (374.25, 194.1084)
  line L1591 (357.75, 194.1084) -> (357.75, 196.4178)
  line L1592 (350.25, 201.9537) -> (352.25, 203.1084)
  line L1593 (358.5, 192.8094) -> (356.5, 191.6547)
  line L1594 (383.25, 219.9537) -> (385.25, 221.1084)
  line L1595 (372.25, 215.5725) -> (370.25, 214.4178)
  line L1596 (362, 243.3453) -> (364, 242.1906)
  line L1597 (349.7943, 193.2169) -> (350.25, 192.9537)
  line L1598 (373, 216.3453) -> (375, 215.1906)
  line L1599 (353.75, 194.1084) -> (355.75, 192.9537)
  line L1600 (408, 228.8094) -> (406, 227.6547)
  line L1601 (390.75, 194.1084) -> (390.75, 196.4178)
  line L1602 (364, 228.8094) -> (362, 227.6547)
  line L1603 (350.25, 197.5725) -> (348.25, 196.4178)
  line L1604 (383.25, 219.9537) -> (385.25, 221.1084)
  line L1605 (372.25, 192.9537) -> (374.25, 194.1084)
  line L1606 (381.25, 221.1084) -> (383.25, 219.9537)
  line L1607 (360.5, 191.6547) -> (358.5, 192.8094)
  line L1608 (350.25, 201.9537) -> (352.25, 203.1084)
  line L1609 (385.25, 194.1084) -> (385.25, 196.4178)
  line L1610 (388.75, 201.9537) -> (390.75, 203.1084)
  line L1611 (352.25, 196.4178) -> (350.25, 197.5725)
  line L1612 (362, 225.3453) -> (364, 224.1906)
  line L1613 (385.25, 194.1084) -> (385.25, 196.4178)
  line L1614 (403.25, 232.4178) -> (403.25, 230.1084)
  line L1615 (405.25, 228.9537) -> (407.25, 230.1084)
  line L1616 (367.5, 198.3453) -> (369.5, 197.1906)
  line L1617 (353.75, 203.1084) -> (355.75, 201.9537)
  line L1618 (395, 227.6547) -> (395, 225.3453)
  line L1619 (357.75, 196.4178) -> (355.75, 197.5725)
  line L1620 (371.5, 198.3453) -> (371.5, 200.6547)
  line L1621 (370.25, 221.1084) -> (372.25, 219.9537)
  line L1622 (369.5, 192.8094) -> (367.5, 191.6547)
  line L1623 (369.5, 201.8094) -> (367.5, 200.6547)
  line L1624 (397.75, 241.4178) -> (397.75, 239.1084)
  line L1625 (397, 228.8094) -> (395, 227.6547)
  line L1626 (384, 198.3453) -> (386, 197.1906)
  line L1627 (374.25, 196.4178) -> (372.25, 197.5725)
  line L1628 (361.25, 219.9537) -> (363.25, 221.1084)
  line L1629 (388, 200.6547) -> (386, 201.8094)
  line L1630 (364, 237.8094) -> (362, 236.6547)
  line L1631 (374.25, 214.4178) -> (372.25, 215.5725)
  line L1632 (373, 198.3453) -> (375, 197.1906)
  line L1633 (369.5, 197.1906) -> (371.5, 198.3453)
  line L1634 (397, 233.1906) -> (399, 234.3453)
  line L1635 (388.75, 197.5725) -> (386.75, 196.4178)
  line L1636 (355.75, 192.9537) -> (357.75, 194.1084)
  line L1637 (372.25, 215.5725) -> (370.25, 214.4178)
  line L1638 (375, 192.8094) -> (373, 191.6547)
  line L1639 (373, 200.6547) -> (373, 198.3453)
  line L1640 (372.25, 201.9537) -> (374.25, 203.1084)
  line L1641 (371.5, 191.6547) -> (369.5, 192.8094)
  line L1642 (350.25, 197.5725) -> (348.25, 196.4178)
  line L1643 (359.25, 196.4178) -> (359.25, 194.1084)
  line L1644 (362, 243.3453) -> (364, 242.1906)
  line L1645 (375, 219.8094) -> (373, 218.6547)
  line L1646 (397.75, 241.4178) -> (397.75, 239.1084)
  line L1647 (384, 200.6547) -> (384, 198.3453)
  line L1648 (355.75, 197.5725) -> (353.75, 196.4178)
  line L1649 (367.5, 198.3453) -> (369.5, 197.1906)
  line L1650 (373, 200.6547) -> (373, 198.3453)
  line L1651 (372.25, 219.9537) -> (374.25, 221.1084)
  line L1652 (349.5, 198.3453) -> (349.5, 200.6547)
  line L1653 (369.5, 201.8094) -> (367.5, 200.6547)
  line L1654 (361.25, 228.9537) -> (363.25, 230.1084)
  arc A56 (401.75, 240.0707) -> (399.5428, 242.4529) centre (375, 217.5) ccw
  line L1655 (374.25, 194.1084) -> (374.25, 196.4178)
  line L1656 (369.5, 197.1906) -> (371.5, 198.3453)
  line L1657 (364, 219.8094) -> (362, 218.6547)
  arc A57 (401.75, 240.0707) -> (399.5428, 242.4529) centre (375, 217.5) ccw
  line L1658 (371.5, 191.6547) -> (369.5, 192.8094)
  line L1659 (381.25, 221.1084) -> (383.25, 219.9537)
  line L1660 (391.5, 201.8094) -> (389.5, 200.6547)
  line L1661 (388.75, 201.9537) -> (390.75, 203.1084)
  line L1662 (396.25, 239.1084) -> (396.25, 241.4178)
  line L1663 (371.5, 200.6547) -> (369.5, 201.8094)
  line L1664 (389.5, 198.3453) -> (391.5, 197.1906)
  line L1665 (375.75, 221.1084) -> (377.75, 219.9537)
  line L1666 (362, 216.3453) -> (364, 215.1906)
  line L1667 (370.25, 196.4178) -> (370.25, 194.1084)
  line L1668 (386.75, 196.4178) -> (386.75, 194.1084)
  line L1669 (362, 207.3453) -> (364, 206.1906)
  line L1670 (374.25, 194.1084) -> (374.25, 196.4178)
  line L1671 (390.75, 239.1084) -> (390.75, 241.4178)
  line L1672 (358.5, 201.8094) -> (356.5, 200.6547)
  line L1673 (370.25, 194.1084) -> (372.25, 192.9537)
  line L1674 (396.25, 239.1084) -> (396.25, 241.4178)
  line L1675 (384, 200.6547) -> (384, 198.3453)
  line L1676 (386.75, 221.1084) -> (388.75, 219.9537)
  line L1677 (363.25, 223.4178) -> (361.25, 224.5725)
  line L1678 (390.75, 194.1084) -> (390.75, 196.4178)
  line L1679 (370.25, 203.1084) -> (372.25, 201.9537)
  line L1680 (364, 210.8094) -> (362, 209.6547)
  line L1681 (396.25, 241.4178) -> (394.25, 242.5725)
  line L1682 (396.25, 232.4178) -> (394.25, 233.5725)
  line L1683 (371.5, 200.6547) -> (369.5, 201.8094)
  line L1684 (391.5, 201.8094) -> (389.5, 200.6547)
  line L1685 (386, 197.1906) -> (388, 198.3453)
  line L1686 (375, 201.8094) -> (373, 200.6547)
  line L1687 (373, 225.3453) -> (375, 224.1906)
  line L1688 (392.25, 241.4178) -> (392.25, 239.1084)
  line L1689 (371.5, 198.3453) -> (371.5, 200.6547)
  line L1690 (394.25, 228.9537) -> (396.25, 230.1084)
  line L1691 (400.5, 207.3453) -> (402.5, 206.1906)
  line L1692 (402.5, 197.1906) -> (404.1665, 198.1527)
  line L1693 (405.25, 210.9537) -> (407.25, 212.1084)
  line L1694 (403.25, 212.1084) -> (405.25, 210.9537)
  line L1695 (378.5, 191.6547) -> (378.5, 189.3453)
  line L1696 (388, 189.3453) -> (388, 191.6547)
  line L1697 (386, 188.1906) -> (388, 189.3453)
  line L1698 (377, 189.3453) -> (377, 191.6547)
  line L1699 (384, 191.6547) -> (384, 189.3453)
  line L1700 (378.5, 189.3453) -> (380.5, 188.1906)
  line L1701 (382.5, 189.3453) -> (382.5, 191.6547)
  line L1702 (385.25, 187.4178) -> (383.25, 188.5725)
  line L1703 (384, 189.3453) -> (386, 188.1906)
  line L1704 (383.25, 188.5725) -> (381.25, 187.4178)
  line L1705 (379.75, 187.4178) -> (377.75, 188.5725)
  line L1706 (377.75, 188.5725) -> (375.75, 187.4178)
  line L1707 (385.25, 187.4178) -> (383.25, 188.5725)
  line L1708 (378.5, 189.3453) -> (380.5, 188.1906)
  line L1709 (383.25, 188.5725) -> (381.25, 187.4178)
  line L1710 (382.5, 189.3453) -> (382.5, 191.6547)
  line L1711 (377, 189.3453) -> (377, 191.6547)
  line L1712 (378.5, 191.6547) -> (378.5, 189.3453)
  line L1713 (384, 191.6547) -> (384, 189.3453)
  line L1714 (377.75, 188.5725) -> (375.75, 187.4178)
  line L1715 (403.25, 212.1084) -> (405.25, 210.9537)
  arc A58 (409.5109, 211.6691) -> (409.917, 215.0916) centre (375, 217.5) ccw
  line L1716 (408.75, 212.1084) -> (409.5109, 211.6691)
  line L1717 (408.75, 214.4178) -> (408.75, 212.1084)
  line L1718 (409.917, 215.0916) -> (408.75, 214.4178)
  line L1719 (409.211, 210.1102) -> (408, 210.8094)
  line L1720 (407.25, 212.1084) -> (407.25, 214.4178)
  line L1721 (408.75, 212.1084) -> (409.5109, 211.6691)
  line L1722 (403.25, 214.4178) -> (403.25, 212.1084)
  line L1723 (408.75, 214.4178) -> (408.75, 212.1084)
  line L1724 (408, 210.8094) -> (406, 209.6547)
  arc A59 (378.5436, 182.6798) -> (381.6602, 183.1395) centre (375, 217.5) ccw
  line L1725 (386.75, 185.1084) -> (387.3612, 184.7555)
  line L1726 (386.75, 185.1084) -> (387.3612, 184.7555)
  line L1727 (375.75, 185.1084) -> (377.75, 183.9537)
  line L1728 (377.75, 183.9537) -> (379.75, 185.1084)
  line L1729 (383.25, 183.9537) -> (385.25, 185.1084)
  line L1730 (377, 182.5572) -> (377, 182.6547)
  line L1731 (383.25, 183.9537) -> (385.25, 185.1084)
  arc A60 (378.5436, 182.6798) -> (381.6602, 183.1395) centre (375, 217.5) ccw
  line L1732 (380.5, 183.8094) -> (378.5436, 182.6798)
  line L1733 (377, 182.5572) -> (377, 182.6547)
  line L1734 (381.6602, 183.1395) -> (380.5, 183.8094)
  line L1735 (380.5, 183.8094) -> (378.5436, 182.6798)
  line L1736 (377.75, 183.9537) -> (379.75, 185.1084)
  line L1737 (381.25, 185.1084) -> (383.25, 183.9537)
  line L1738 (375.75, 185.1084) -> (377.75, 183.9537)
  line L1739 (381.25, 185.1084) -> (383.25, 183.9537)
  line L1740 (381.6602, 183.1395) -> (380.5, 183.8094)
  line L1741 (353.75, 212.1084) -> (355.75, 210.9537)
  line L1742 (374.25, 223.4178) -> (372.25, 224.5725)
  line L1743 (388, 200.6547) -> (386, 201.8094)
  line L1744 (386, 201.8094) -> (384, 200.6547)
  line L1745 (399.75, 228.9537) -> (401.75, 230.1084)
  line L1746 (393.5, 243.3453) -> (393.5, 245.6547)
  line L1747 (374.25, 212.1084) -> (374.25, 214.4178)
  line L1748 (384, 225.3453) -> (386, 224.1906)
  line L1749 (402.5, 228.8094) -> (400.5, 227.6547)
  line L1750 (374.25, 230.1084) -> (374.25, 232.4178)
  line L1751 (363.25, 194.1084) -> (363.25, 196.4178)
  line L1752 (374.25, 230.1084) -> (374.25, 232.4178)
  line L1753 (369.5, 192.8094) -> (367.5, 191.6547)
  arc A61 (398.7552, 243.2039) -> (395.442, 245.9099) centre (375, 217.5) ccw
  line L1754 (370.25, 214.4178) -> (370.25, 212.1084)
  line L1755 (399.75, 233.5725) -> (397.75, 232.4178)
  line L1756 (386, 224.1906) -> (388, 225.3453)
  line L1757 (362, 200.6547) -> (362, 198.3453)
  line L1758 (391.5, 228.8094) -> (389.5, 227.6547)
  line L1759 (385.25, 203.1084) -> (385.25, 205.4178)
  line L1760 (396.25, 232.4178) -> (394.25, 233.5725)
  line L1761 (391.5, 228.8094) -> (389.5, 227.6547)
  line L1762 (399.75, 228.9537) -> (401.75, 230.1084)
  line L1763 (388.75, 192.9537) -> (390.75, 194.1084)
  line L1764 (388.75, 224.5725) -> (386.75, 223.4178)
  line L1765 (397, 233.1906) -> (399, 234.3453)
  line L1766 (374.25, 232.4178) -> (372.25, 233.5725)
  line L1767 (395, 234.3453) -> (397, 233.1906)
  line L1768 (402.5, 228.8094) -> (400.5, 227.6547)
  line L1769 (404.1665, 236.8473) -> (402.5, 237.8094)
  line L1770 (389.5, 200.6547) -> (389.5, 198.3453)
  line L1771 (386.75, 203.1084) -> (388.75, 201.9537)
  line L1772 (401.75, 230.1084) -> (401.75, 232.4178)
  line L1773 (366, 191.6547) -> (364, 192.8094)
  line L1774 (397.75, 232.4178) -> (397.75, 230.1084)
  line L1775 (373, 234.3453) -> (375, 233.1906)
  line L1776 (388.75, 228.9537) -> (390.75, 230.1084)
  line L1777 (379.75, 203.1084) -> (379.75, 205.4178)
  line L1778 (399.75, 233.5725) -> (397.75, 232.4178)
  line L1779 (386.75, 196.4178) -> (386.75, 194.1084)
  line L1780 (379.75, 239.1084) -> (379.75, 241.4178)
  line L1781 (373, 225.3453) -> (375, 224.1906)
  line L1782 (362, 200.6547) -> (362, 198.3453)
  line L1783 (374.25, 223.4178) -> (372.25, 224.5725)
  line L1784 (374.25, 232.4178) -> (372.25, 233.5725)
  line L1785 (397, 228.8094) -> (395, 227.6547)
  line L1786 (372.25, 228.9537) -> (374.25, 230.1084)
  line L1787 (359.25, 223.4178) -> (359.25, 221.1084)
  line L1788 (386.75, 203.1084) -> (388.75, 201.9537)
  line L1789 (379.75, 203.1084) -> (379.75, 205.4178)
  line L1790 (385.25, 239.1084) -> (385.25, 241.4178)
  line L1791 (401.75, 230.1084) -> (401.75, 232.4178)
  line L1792 (388.75, 228.9537) -> (390.75, 230.1084)
  line L1793 (386.75, 241.4178) -> (386.75, 239.1084)
  line L1794 (375.75, 241.4178) -> (375.75, 239.1084)
  line L1795 (375, 228.8094) -> (373, 227.6547)
  line L1796 (367.5, 200.6547) -> (367.5, 198.3453)
  line L1797 (372.25, 224.5725) -> (370.25, 223.4178)
  line L1798 (375.75, 205.4178) -> (375.75, 203.1084)
  line L1799 (358.5, 206.1906) -> (360.5, 207.3453)
  line L1800 (368.75, 212.1084) -> (368.75, 214.4178)
  line L1801 (364, 197.1906) -> (366, 198.3453)
  line L1802 (373, 227.6547) -> (373, 225.3453)
  line L1803 (388, 227.6547) -> (386, 228.8094)
  line L1804 (377.75, 192.9537) -> (379.75, 194.1084)
  line L1805 (392.25, 223.4178) -> (392.25, 221.1084)
  line L1806 (355.75, 206.5725) -> (353.75, 205.4178)
  line L1807 (379.75, 194.1084) -> (379.75, 196.4178)
  line L1808 (357.75, 221.1084) -> (357.75, 223.4178)
  line L1809 (394.25, 237.9537) -> (396.25, 239.1084)
  line L1810 (362, 209.6547) -> (362, 207.3453)
  line L1811 (402.5, 233.1906) -> (404.5, 234.3453)
  line L1812 (386.75, 223.4178) -> (386.75, 221.1084)
  line L1813 (386, 228.8094) -> (384, 227.6547)
  line L1814 (374.25, 221.1084) -> (374.25, 223.4178)
  line L1815 (366.75, 201.9537) -> (368.75, 203.1084)
  line L1816 (364, 201.8094) -> (362, 200.6547)
  line L1817 (356.5, 207.3453) -> (358.5, 206.1906)
  line L1818 (386.75, 205.4178) -> (386.75, 203.1084)
  line L1819 (370.25, 223.4178) -> (370.25, 221.1084)
  line L1820 (374.25, 221.1084) -> (374.25, 223.4178)
  line L1821 (386.75, 241.4178) -> (386.75, 239.1084)
  line L1822 (390.75, 203.1084) -> (390.75, 205.4178)
  line L1823 (370.25, 223.4178) -> (370.25, 221.1084)
  line L1824 (378.5, 200.6547) -> (378.5, 198.3453)
  line L1825 (366.75, 192.9537) -> (368.75, 194.1084)
  line L1826 (358.5, 210.8094) -> (356.5, 209.6547)
  line L1827 (360.5, 209.6547) -> (358.5, 210.8094)
  line L1828 (397.75, 239.1084) -> (399.75, 237.9537)
  line L1829 (392.25, 205.4178) -> (392.25, 203.1084)
  line L1830 (360.5, 209.6547) -> (358.5, 210.8094)
  line L1831 (394.25, 237.9537) -> (396.25, 239.1084)
  line L1832 (388, 227.6547) -> (386, 228.8094)
  line L1833 (360.5, 207.3453) -> (360.5, 209.6547)
  line L1834 (389.5, 227.6547) -> (389.5, 225.3453)
  line L1835 (368.75, 196.4178) -> (366.75, 197.5725)
  line L1836 (385.25, 239.1084) -> (385.25, 241.4178)
  line L1837 (404.5, 227.6547) -> (402.5, 228.8094)
  line L1838 (379.75, 239.1084) -> (379.75, 241.4178)
  line L1839 (377.75, 201.9537) -> (379.75, 203.1084)
  line L1840 (399.75, 237.9537) -> (401.75, 239.1084)
  line L1841 (355, 207.3453) -> (355, 209.6547)
  line L1842 (401.75, 239.1084) -> (401.75, 240.0707)
  line L1843 (363.25, 212.1084) -> (363.25, 214.4178)
  line L1844 (390.75, 223.4178) -> (388.75, 224.5725)
  line L1845 (401.75, 239.1084) -> (401.75, 240.0707)
  line L1846 (385.25, 221.1084) -> (385.25, 223.4178)
  line L1847 (373, 227.6547) -> (373, 225.3453)
  line L1848 (390.75, 203.1084) -> (390.75, 205.4178)
  line L1849 (372.25, 233.5725) -> (370.25, 232.4178)
  line L1850 (370.25, 232.4178) -> (370.25, 230.1084)
  line L1851 (384, 227.6547) -> (384, 225.3453)
  line L1852 (366.75, 201.9537) -> (368.75, 203.1084)
  line L1853 (364, 201.8094) -> (362, 200.6547)
  line L1854 (360.5, 207.3453) -> (360.5, 209.6547)
  line L1855 (364, 192.8094) -> (362, 191.6547)
  line L1856 (367.5, 200.6547) -> (367.5, 198.3453)
  line L1857 (366.75, 192.9537) -> (368.75, 194.1084)
  line L1858 (370.25, 214.4178) -> (370.25, 212.1084)
  line L1859 (363.25, 194.1084) -> (363.25, 196.4178)
  line L1860 (364.75, 214.4178) -> (364.75, 212.1084)
  line L1861 (386.75, 205.4178) -> (386.75, 203.1084)
  line L1862 (379.75, 196.4178) -> (377.75, 197.5725)
  line L1863 (364.75, 196.4178) -> (364.75, 194.1084)
  line L1864 (392.25, 223.4178) -> (392.25, 221.1084)
  line L1865 (375.75, 205.4178) -> (375.75, 203.1084)
  line L1866 (374.25, 212.1084) -> (374.25, 214.4178)
  line L1867 (390.75, 221.1084) -> (390.75, 223.4178)
  line L1868 (366, 200.6547) -> (364, 201.8094)
  line L1869 (364.75, 203.1084) -> (366.75, 201.9537)
  line L1870 (381.25, 241.4178) -> (381.25, 239.1084)
  line L1871 (375.75, 196.4178) -> (375.75, 194.1084)
  line L1872 (366, 198.3453) -> (366, 200.6547)
  line L1873 (375.75, 196.4178) -> (375.75, 194.1084)
  line L1874 (386.75, 230.1084) -> (388.75, 228.9537)
  line L1875 (377, 198.3453) -> (377, 200.6547)
  line L1876 (359.25, 212.1084) -> (361.25, 210.9537)
  line L1877 (375.75, 203.1084) -> (377.75, 201.9537)
  line L1878 (399, 234.3453) -> (399, 236.6547)
  line L1879 (368.75, 194.1084) -> (368.75, 196.4178)
  line L1880 (377.75, 197.5725) -> (375.75, 196.4178)
  line L1881 (397, 237.8094) -> (395, 236.6547)
  line L1882 (382.5, 200.6547) -> (380.5, 201.8094)
  line L1883 (352.25, 221.1084) -> (352.25, 223.4178)
  line L1884 (359.25, 212.1084) -> (361.25, 210.9537)
  line L1885 (361.25, 206.5725) -> (359.25, 205.4178)
  line L1886 (400.5, 234.3453) -> (402.5, 233.1906)
  line L1887 (399, 236.6547) -> (397, 237.8094)
  line L1888 (397.75, 239.1084) -> (399.75, 237.9537)
  line L1889 (348.25, 223.4178) -> (348.25, 221.1084)
  line L1890 (362, 209.6547) -> (362, 207.3453)
  line L1891 (397, 237.8094) -> (395, 236.6547)
  line L1892 (399, 236.6547) -> (397, 237.8094)
  line L1893 (378.5, 198.3453) -> (380.5, 197.1906)
  line L1894 (378.5, 198.3453) -> (380.5, 197.1906)
  line L1895 (366.75, 197.5725) -> (364.75, 196.4178)
  line L1896 (388, 225.3453) -> (388, 227.6547)